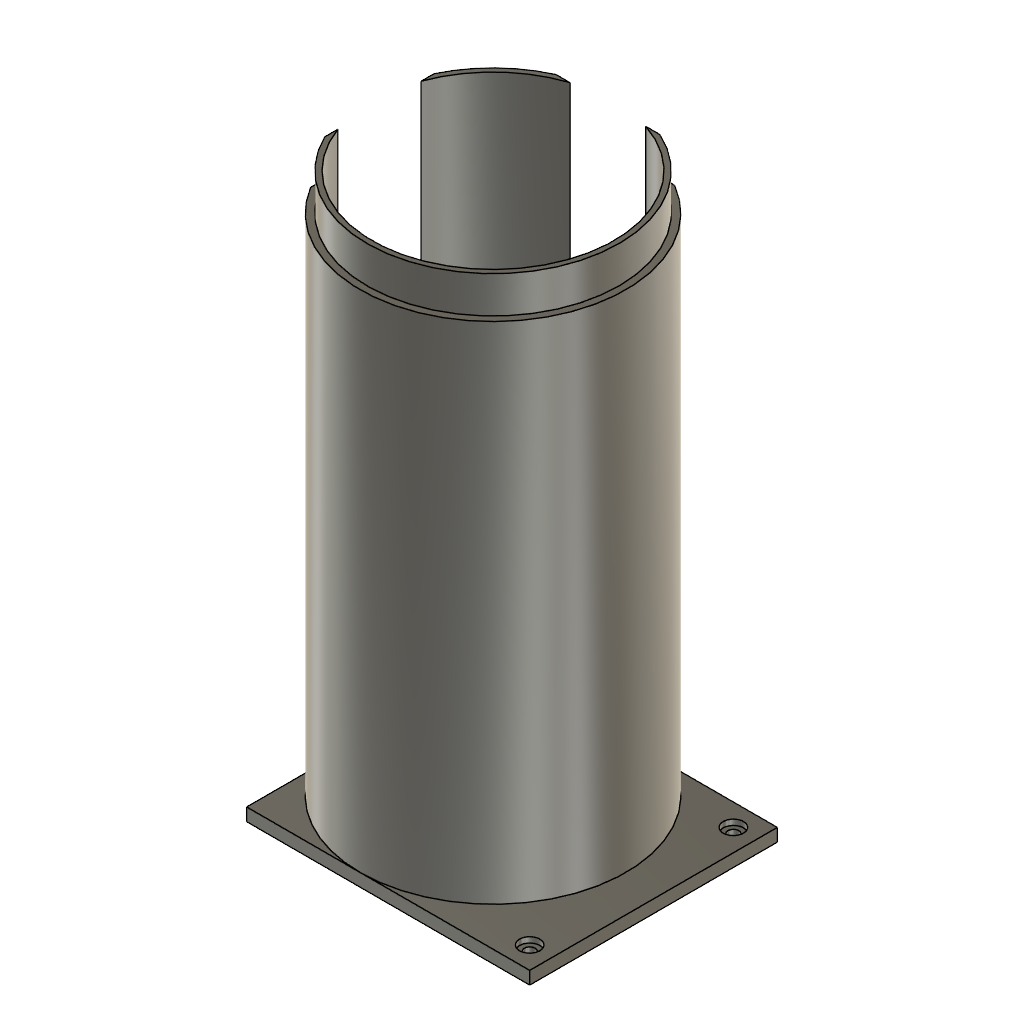
Port Front (Autodesk Fusion 360 design; units mm, degrees)
Autodesk Fusion 360 part; units mm, degrees
sketch "Sketch1" plane through (0, 0, 0) normal (0, 0, 1) x (1, 0, 0)
  circle A0 centre (0, 0) radius 33
  circle A1 centre (0, 0) radius 36.25
  dimension "d1" = 66
  dimension "d2" = 3.25
  constraint coincident A0.centre A1.centre
  measures "d1" diameter of A0
extrude "Extrude1" add sketch "Sketch1" along normal blind 151.205 makes body 1
sketch "Sketch2" plane through (0, 0, 151.205) normal (0, 0, 1) x (-1, 0, 0)
  circle A0 centre (0, 0) radius 33
  circle A1 centre (0, 0) radius 36.25
  circle A2 centre (0, 0) radius 34.75
  dimension "d5" = -1.5
extrude "Extrude2" cut sketch "Sketch2" against normal blind 10 contours A1 bodies 1
sketch "Sketch3" plane through (0, 0, 0) normal (0, 0, -1) x (1, 0, 0)
  circle A0 centre (0, 0) radius 33
  circle A1 centre (0, 0) radius 36.25
  line L0 (0, -33) -> (0, -31.35)
  line L1 (0, -31.35) -> (-18.2, -31.35)
  line L2 (0, -31.35) -> (18.2, -31.35)
  dimension "d8" = 1.65
  constraint coincident A0 L0.start
  constraint vertical L0
  constraint coincident A1 L1.end
  constraint perpendicular L0 L1
  constraint coincident A1 L2.end
  constraint perpendicular L0 L2
  measures "d8" distance of L0.start L0.end
extrude "Extrude3" cut sketch "Sketch3" against normal blind 158 contours A0 L0 L1 | A0 A1 L1 L2 | A0 L0 L2 picked at (11.2202, -33.2731) bodies 1
sketch "Sketch4" plane through (0, 0, 151.205) normal (0, 0, 1) x (-1, 0, 0)
  line L0 (10.3042, -31.35) -> (14.9913, -31.35)
  arc A0 (14.9913, -31.35) -> (-14.9913, -31.35) centre (0, 0) ccw
  line L1 (-14.9913, -31.35) -> (-10.3042, -31.35)
  arc A1 (10.3042, -31.35) -> (-10.3042, -31.35) centre (0, 0) ccw
  arc A2 (10.3042, -31.35) -> (-10.3042, -31.35) centre (0, 0) ccw
  line L2 (0, 33) -> (34.4605, 33)
  constraint midpoint A2 L2.start
  constraint tangent A1 L2
  constraint horizontal L2
sketch "Sketch5" plane through (0, 0, 0) normal (0, 0, -1) x (1, 0, 0)
  line L0 (-18.2, -31.35) -> (-10.3042, -31.35)
  arc A0 (10.3042, -31.35) -> (-10.3042, -31.35) centre (0, 0) ccw
  line L1 (10.3042, -31.35) -> (18.2, -31.35)
  arc A1 (18.2, -31.35) -> (-18.2, -31.35) centre (0, 0) ccw
  line L2 (-36.25, 0) -> (-36.25, -31.35)
  line L3 (-36.25, -31.35) -> (-18.2, -31.35)
  line L4 (36.25, 0) -> (36.25, -31.35)
  line L5 (36.25, -31.35) -> (18.2, -31.35)
  line L6 (-36.25, 0) -> (-36.25, 36.25)
  line L7 (36.25, 0) -> (36.25, 36.25)
  line L8 (36.25, 36.25) -> (-36.25, 36.25)
  line L9 (-36.25, 36.25) -> (-46.25, 36.25)
  line L10 (-46.25, 36.25) -> (-46.25, -31.35)
  line L11 (-46.25, -31.35) -> (-36.25, -31.35)
  line L12 (-36.25, -31.35) -> (-36.25, 36.25)
  line L13 (36.25, 36.25) -> (46.25, 36.25)
  line L14 (46.25, 36.25) -> (46.25, -31.35)
  line L15 (46.25, -31.35) -> (36.25, -31.35)
  line L16 (36.25, -31.35) -> (36.25, 36.25)
  dimension "d13" = 10
  dimension "d14" = 10
  constraint coincident A1 L2.start
  constraint tangent A1 L2
  constraint perpendicular L1 L2
  constraint coincident L0.start A1.end
  constraint perpendicular L2 L3
  constraint coincident A1 L4.start
  constraint tangent A1 L4
  constraint perpendicular L3 L4
  constraint coincident L1.end A1.start
  constraint perpendicular L4 L5
  constraint tangent A1 L6
  constraint tangent A1 L7
  constraint perpendicular L6 L8
  constraint horizontal L9
  constraint vertical L10
  constraint horizontal L11
  constraint vertical L12
  constraint horizontal L13
  constraint vertical L14
  constraint horizontal L15
  constraint vertical L16
  measures "d13" distance of L6.end L9.end
  measures "d14" distance of L7.end L13.end
extrude "Extrude4" add sketch "Sketch5" against normal blind 3.5 contours A1 L2 L3 L12 | A1 L6 L8 L12 | L2 L6 L9 L10 L11 L12 | A1 L7 L8 L16 | A1 L4 L5 L16 | L4 L7 L13 L14 L15 L16 bodies 1
sketch "Sketch6" plane through (0, 0, 3.5) normal (0, 0, 1) x (-1, 0, 0)
  line L0 (46.25, 36.25) -> (0, 36.25)
  arc A0 (18.2, -31.35) -> (0, 36.25) centre (0, 0) ccw
  line L1 (18.2, -31.35) -> (46.25, -31.35)
  line L2 (46.25, -31.35) -> (46.25, 36.25)
  line L3 (46.25, -31.35) -> (40.2396, -25.3396)
  line L4 (46.25, -31.35) -> (54.75, -31.35) construction
  circle A1 centre (40.2396, -25.3396) radius 1.475
  line L5 (46.25, 36.25) -> (40.2396, 30.2396)
  line L6 (46.25, 36.25) -> (54.75, 36.25) construction
  circle A2 centre (40.2396, 30.2396) radius 1.475
  line L7 (0, 36.25) -> (0, 41.3263)
  circle A3 centre (-40.2396, 30.2396) radius 1.475
  circle A4 centre (-40.2396, -25.3396) radius 1.475
  dimension "d15" = 135
  dimension "d16" = 8.5
  dimension "d17" = 2.95
  dimension "d18" = 135
  dimension "d19" = 8.5
  dimension "d20" = 2.95
  constraint horizontal L4
  constraint coincident L1.end L2.start
  constraint coincident L3.end A1.centre
  constraint horizontal L6
  constraint coincident L0.start L2.end
  constraint coincident L5.end A2.centre
  constraint coincident L0.end A0.end
  constraint perpendicular L0 L7
  constraint symmetric A1 L7 A4
  constraint symmetric A2 L7 A3
  measures "d15" angle of L3 L4
  measures "d16" distance of L1.end L3.end
  measures "d17" diameter of A1
  measures "d18" angle of L5 L6
  measures "d19" distance of L0.start L5.end
  measures "d20" diameter of A2
extrude "Extrude5" cut sketch "Sketch6" against normal blind 25 contours A1 | A2 | A3 | A4 bodies 1
sketch "Sketch7" plane through (0, 0, 3.5) normal (0, 0, 1) x (-1, 0, 0)
  circle A0 centre (40.2396, -25.3396) radius 1.475
  circle A1 centre (40.2396, 30.2396) radius 1.475
  line L0 (46.25, 36.25) -> (0, 36.25)
  arc A2 (18.2, -31.35) -> (0, 36.25) centre (0, 0) ccw
  line L1 (18.2, -31.35) -> (46.25, -31.35)
  line L2 (46.25, -31.35) -> (46.25, 36.25)
  circle A3 centre (40.2396, -25.3396) radius 2.775
  circle A4 centre (40.2396, 30.2396) radius 2.775
  line L3 (0, 36.25) -> (0, 42.0479)
  circle A5 centre (-40.2396, 30.2396) radius 2.775
  circle A6 centre (-40.2396, -25.3396) radius 2.775
  dimension "d23" = 5.55
  dimension "d24" = 5.55
  constraint concentric A0 A3
  constraint concentric A1 A4
  constraint coincident L0.end A2.end
  constraint perpendicular L0 L3
  constraint symmetric A3 L3 A6
  constraint symmetric A4 L3 A5
  measures "d23" diameter of A3
  measures "d24" diameter of A4
extrude "Extrude6" cut sketch "Sketch7" against normal blind 1.5 contours A3 | A4 | A5 | A6 bodies 1
extrude "Extrude7" cut 1 faces at (-13.3762, 30.7261, 151.205) along direction (0, 0, -1) blind 10 on bodies 1 bodies 1
sketch "Sketch8" plane through (0, 0, 141.205) normal (0, 0, 1) x (-1, 0, 0)
  line L0 (10.3042, -31.35) -> (18.2, -31.35)
  arc A0 (18.2, -31.35) -> (-18.2, -31.35) centre (0, 0) ccw
  line L1 (-18.2, -31.35) -> (-10.3042, -31.35)
  arc A1 (10.3042, -31.35) -> (-10.3042, -31.35) centre (0, 0) ccw
  circle A2 centre (0, 0) radius 33
  circle A3 centre (0, 0) radius 34.4
  line L2 (10.3042, -31.35) -> (14.2521, -31.35)
  line L3 (-10.3042, -31.35) -> (-14.2521, -31.35)
  dimension "d29" = 1.4
  constraint concentric A0 A2
  constraint coincident L0.start A1.start
  constraint midpoint L0 L2.end
  constraint coincident L1.end A1.end
  constraint midpoint L1 L3.end
extrude "Extrude8" add sketch "Sketch8" along normal blind 10 contours L0 L1 A1 A2 A3 L2 L3 bodies 1
sketch "Sketch9" plane through (0, 0, 0) normal (0, 0, -1) x (1, 0, 0)
  circle A0 centre (40.2396, -25.3396) radius 1.475
  circle A1 centre (-40.2396, -25.3396) radius 1.475
  circle A2 centre (40.2396, 30.2396) radius 1.475
  circle A3 centre (-40.2396, 30.2396) radius 1.475
  line L0 (-46.25, -31.35) -> (-10.3042, -31.35)
  arc A4 (10.3042, -31.35) -> (-10.3042, -31.35) centre (0, 0) ccw
  line L1 (10.3042, -31.35) -> (46.25, -31.35)
  line L2 (46.25, -31.35) -> (46.25, 36.25)
  line L3 (46.25, 36.25) -> (-46.25, 36.25)
  line L4 (-46.25, 36.25) -> (-46.25, -31.35)
  line L5 (-33, 0) -> (-31, 0)
  line L6 (-31, 0) -> (-31, 42.6088)
  line L7 (-31, 42.6088) -> (-54.7973, 42.6088)
  line L8 (-54.7973, 42.6088) -> (-54.7973, -36.6322)
  line L9 (-54.7973, -36.6322) -> (-31, -36.6322)
  line L10 (-31, -36.6322) -> (-31, 0)
  dimension "d32" = 2
  constraint coincident A4 L5.start
  constraint horizontal L5
  constraint perpendicular L3 L6
  constraint perpendicular L6 L7
  constraint perpendicular L7 L8
  constraint perpendicular L8 L9
  constraint perpendicular L5 L10
  measures "d32" distance of L5.start L5.end
extrude "Extrude9" cut sketch "Sketch9" against normal blind 155 contours A1 | A3 | L0 A4 L3 L4 L6 L10 | L0 L3 L4 L6 L7 L8 L9 L10 | A4 L5 L10 | A4 L5 L6 bodies 1 makes body 2 at (-20.2765, 26.0358, 50.4017)
